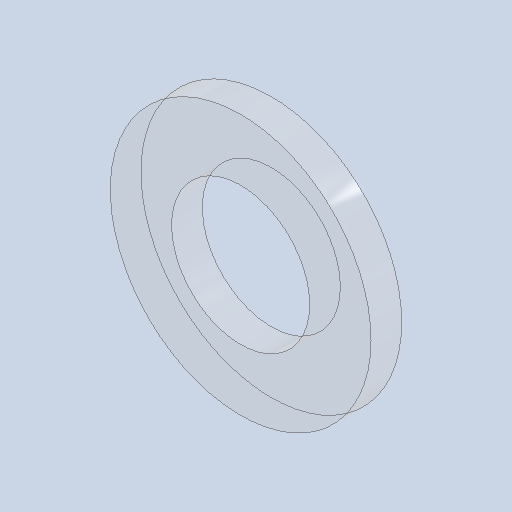
# Autodesk Inventor part: АНЦП.014.00.00.006
Saved by Autodesk Inventor 2022 (Build 260153000, 153)
## iProperties
Created: 2022-02-10
Part Number: АНЦП.014.00.00.006
Material: PET Plastic
Document SubType Name: Modeling
Designer: br4ch
Density: 1.541 g/cm^3
Appearance: Polycarbonate - Clear
Mass: 0.503484 g
Surface Area: 4.90088 cm^2
Volume: 0.326726 cm^3
Author: br4ch
Autodesk Inventor part; units mm, degrees
ref_plane "YZ Plane" through (0, 0, 0) normal (1, 0, 0) x (0, 1, 0)
ref_plane "XZ Plane" through (0, 0, 0) normal (0, 1, 0) x (-1, 0, 0)
ref_plane "XY Plane" through (0, 0, 0) normal (0, 0, 1) x (1, 0, 0)
sketch "Sketch1" plane through (0, 0, 0) normal (0, 0, 1) x (1, 0, 0)
  circle A0 centre (0, 0) radius 8.5
  circle A1 centre (0, 0) radius 4.5
  dimension "d0" = 17
  dimension "d1" = 9
  constraints: 2 centre point, 2 coincident
  measures "d0" diameter of A0
  measures "d1" diameter of A1
extrude "Extrusion1" add sketch "Sketch1" along normal blind 2
body "Solid1"
